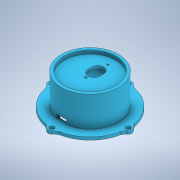
# Autodesk Inventor part: Pieza1parte3
Saved by Autodesk Inventor 2021 (Build 250183000, 183)
## iProperties
Created: 2021-03-28
Part Number: Pieza1parte3
Material: Genérico
Document SubType Name: Modeling
Designer: Arturo
Density: 1 g/cm^3
Appearance: Valor por defecto
Author: Arturo
Autodesk Inventor part; units mm, degrees
ref_plane "YZ Plane" through (0, 0, 0) normal (1, 0, 0) x (0, 1, 0)
ref_plane "XZ Plane" through (0, 0, 0) normal (0, 1, 0) x (-1, 0, 0)
ref_plane "XY Plane" through (0, 0, 0) normal (0, 0, 1) x (1, 0, 0)
sketch "Boceto1" plane through (0, 0, 0) normal (0, 1, 0) x (-1, 0, 0)
  line L0 (0, 0) -> (12.5, 0)
  line L1 (12.5, 0) -> (12.5, -5)
  line L2 (0, -5) -> (0, 0)
  circle A0 centre (6.25, -2.5) radius 1
  arc A1 (8.4861, -5) -> (4.0139, -5) centre (6.25, -7) ccw
  line L3 (12.5, -5) -> (8.4861, -5)
  line L4 (4.0139, -5) -> (0, -5)
  dimension "d1" = 5
  dimension "d2" = 2
  dimension "d4" = 6
  constraints: 10 end point, 3 parallel, 2 centre point, 2 point on circle, 1 horizontal, 1 perpendicular
  measures "d1" distance of L0.end L1.end
  measures "d2" diameter of A0
  measures "d4" diameter of A1
extrude "Extrusión1" add sketch "Boceto1" along normal blind 5
sketch "Boceto2" plane through (0, 5, 0) normal (0, 1, 0) x (1, 0, 0)
  line L0 (0, 5) -> (-4.0139, 5) projected
  arc A0 (-8.4861, 5) -> (-4.0139, 5) centre (-6.25, 7) ccw projected
  line L1 (-8.4861, 5) -> (-12.5, 5) projected
  line L2 (-12.5, 5) -> (-12.5, 0) projected
  line L3 (-12.5, 0) -> (0, 0) projected
  line L4 (0, 0) -> (0, 5) projected
  circle A1 centre (-6.25, 2.5) radius 1 projected
  arc A2 (-12.5, 11.25) -> (0, 11.25) centre (-6.25, 11.25) ccw
  arc A3 (0, 15.25) -> (-12.5, 15.25) centre (-6.25, 15.25) ccw
  line L5 (-12.5, 11.25) -> (-12.5, 15.25)
  line L6 (0, 11.25) -> (0, 15.25)
  line L7 (0, 23.25) -> (-12.5, 23.25)
  line L8 (-12.5, 23.25) -> (-12.5, 28.25)
  line L9 (-12.5, 28.25) -> (0, 28.25)
  line L10 (0, 28.25) -> (0, 23.25)
  circle A4 centre (-6.25, 25.75) radius 1
  circle A5 centre (-6.25, 7) radius 27
  circle A6 centre (-6.25, 7) radius 30
  dimension "d8" = 12.5
  dimension "d10" = 12.5
  dimension "d12" = 12.5
  dimension "d13" = 5
  dimension "d14" = 2
  dimension "d15" = 54
  dimension "d17" = 3
  constraints: 12 end point, 5 centre point, 4 point on circle, 2 coincident, 2 parallel, 2 tangent, 1 horizontal, 1 perpendicular
  measures "d8" diameter of A2
  measures "d10" diameter of A3
  measures "d12" distance of L8.end L9.end
  measures "d13" distance of L7.end L8.end
  measures "d14" diameter of A4
  measures "d15" diameter of A5
  measures "d17" radial gap between concentric circles of A5 A6
extrude "Extrusión2" add sketch "Boceto2" along normal blind 3 contours A5
extrude "Extrusión3" add sketch "Boceto2" against normal blind 5 contours L7 L8 L9 L10
extrude "Extrusión4" add sketch "Boceto2" along normal blind 6.8 contours A6
sketch "Boceto3" plane through (0, 5, 0) normal (0, 1, 0) x (1, 0, 0)
  line L0 (-4.0139, 5) -> (0, 5) projected
  line L1 (0, 0) -> (-12.5, 0) projected
  line L2 (0, 5) -> (-12.5, 5)
  line L3 (-12.5, 5) -> (-12.5, 0)
  line L4 (-12.5, 0) -> (0, 0)
  line L5 (0, 0) -> (0, 5)
  line L6 (-12.5, 28.25) -> (0, 28.25) projected
  line L7 (0, 23.25) -> (-12.5, 23.25) projected
  line L8 (0, 28.25) -> (-12.5, 28.25)
  line L9 (-12.5, 28.25) -> (-12.5, 23.25)
  line L10 (-12.5, 23.25) -> (0, 23.25)
  line L11 (0, 23.25) -> (0, 28.25)
  circle A0 centre (-6.25, 25.75) radius 1 projected
  circle A1 centre (-6.25, 25.75) radius 1
  circle A2 centre (-6.25, 2.5) radius 1 projected
  circle A3 centre (-6.25, 2.5) radius 1
  dimension "d24" = 12.5
  dimension "d25" = 5
  dimension "d26" = 12.5
  dimension "d27" = 5
  dimension "d28" = 2
  dimension "d29" = 2
  constraints: 16 end point, 4 parallel, 2 centre point, 2 coincident, 2 horizontal, 2 perpendicular
  measures "d24" distance of L4.end L1.end
  measures "d25" distance of L1.end L2.end
  measures "d26" distance of L10.end L7.end
  measures "d27" distance of L7.end L8.end
  measures "d28" diameter of A1
  measures "d29" diameter of A3
extrude "Extrusión5" add sketch "Boceto3" along normal blind 3
sketch "Boceto4" plane through (-6.25, 5, -7) normal (0, -1, 0) x (1, 0, 0)
  circle A0 centre (0, 0) radius 27 projected
  circle A1 centre (0, 0) radius 30
  circle A2 centre (0, 0) radius 27
  point P0 (6.25, 7)
  dimension "d32" = 60
  dimension "d33" = 54
  constraints: 2 centre point, 2 coincident
  measures "d32" diameter of A1
  measures "d33" diameter of A2
extrude "Extrusión6" add sketch "Boceto4" along normal blind 25
sketch "Boceto5" plane through (-6.25, -20, -7) normal (0, -1, 0) x (1, 0, 0)
  circle A0 centre (0, 0) radius 27 projected
  arc A1 (6.25, -4.25) -> (-6.25, -4.25) centre (0, -4.25) ccw projected
  line L0 (6.25, -8.25) -> (6.25, -4.25) projected
  arc A2 (-6.25, -8.25) -> (6.25, -8.25) centre (0, -8.25) ccw projected
  line L1 (-6.25, -4.25) -> (-6.25, -8.25) projected
  arc A3 (2.2361, 2) -> (-2.2361, 2) centre (0, 0) ccw projected
  line L2 (-2.2361, 2) -> (-6.25, 2) projected
  line L3 (-6.25, 2) -> (-6.25, 7) projected
  line L4 (-6.25, 7) -> (6.25, 7) projected
  line L5 (6.25, 7) -> (6.25, 2) projected
  line L6 (6.25, 2) -> (2.2361, 2) projected
  line L7 (6.25, -16.25) -> (-6.25, -16.25) projected
  line L8 (6.25, -21.25) -> (6.25, -16.25) projected
  line L9 (-6.25, -21.25) -> (6.25, -21.25) projected
  line L10 (-6.25, -16.25) -> (-6.25, -21.25) projected
  circle A4 centre (0, 0) radius 30 projected
  circle A5 centre (0, 0) radius 27 projected
  circle A6 centre (0, 0) radius 40
  circle A7 centre (0, 0) radius 30 projected
  line L11 (0, 30) -> (5, 30)
  line L12 (5, 30) -> (-5, 30)
  line L13 (-5, 30) -> (-5, 26.533)
  circle A8 centre (0, 0) radius 27 projected
  line L14 (5, 30) -> (5, 26.533)
  circle A9 centre (0, 0) radius 27
  circle A10 centre (0, 0) radius 30
  dimension "d36" = 80
  dimension "d37" = 5
  dimension "d38" = 10
  constraints: 8 end point, 3 centre point, 3 coincident, 2 horizontal, 2 point on circle, 1 concentric, 1 parallel, 1 perpendicular, 1 point on line, 1 vertical alignment, 2 other
  measures "d36" diameter of A6
  measures "d37" distance of L11.start L11.end
  measures "d38" distance of L11.end L12.end
extrude "Extrusión7" add sketch "Boceto5" along normal blind 3 contours A0 L14 A4 L13 | A0 L13 A4 L14 | A4 L11 L14 | L13 L12 A4 | A6
sketch "Boceto6" plane through (-6.25, -23, -7) normal (0, -1, 0) x (1, 0, 0)
  circle A0 centre (0, 0) radius 30 projected
  circle A1 centre (0, 0) radius 40 projected
  circle A2 centre (0, 0) radius 27 projected
  circle A3 centre (0, 0) radius 30 projected
  circle A4 centre (0, 0) radius 30 projected
  circle A5 centre (0, 0) radius 40 projected
  arc A6 (42.4961, -3.1256) -> (42.4568, 3.1566) centre (40, 0) ccw
  circle A7 centre (40, 0) radius 2.5
  circle A8 centre (0, 0) radius 40
  arc A9 (42.4961, -3.1256) -> (39.2164, -7.8789) centre (48.7365, -10.9396) ccw
  line L0 (39.8, 3.995) -> (39.8, 3.995)
  arc A10 (39.3287, 7.2975) -> (42.4568, 3.1566) centre (48.5987, 11.0482) ccw
  arc A11 (3.1545, 42.4596) -> (-3.1252, 42.4966) centre (0, 40) ccw
  circle A12 centre (0, 40) radius 2.5
  line L1 (3.995, 39.8) -> (3.995, 39.8)
  line L2 (9.1155, 38.7955) -> (7.182, 39.1748)
  arc A13 (3.1545, 42.4596) -> (9.1155, 38.7955) centre (11.0406, 48.6084) ccw
  line L3 (-3.995, 39.8) -> (-3.995, 39.8)
  line L4 (-9.2166, 38.8873) -> (-9.7422, 38.7955)
  arc A14 (-9.2166, 38.8873) -> (-3.1252, 42.4966) centre (-10.9383, 48.738) ccw
  arc A15 (-3.2297, -42.3598) -> (3.1372, -42.4816) centre (0, -40) ccw
  circle A16 centre (0, -40) radius 2.5
  arc A17 (-42.4596, 3.1545) -> (-42.4753, -3.1421) centre (-40, 0) ccw
  circle A18 centre (-40, 0) radius 2.5
  line L5 (-8.8392, -38.5679) -> (-8.6091, -38.6265)
  arc A19 (7.6163, -39.2682) -> (3.1372, -42.4816) centre (10.9801, -48.6855) ccw
  arc A20 (-3.2297, -42.3598) -> (-6.5544, -39.4593) centre (-11.3041, -48.2594) ccw
  arc A21 (-42.4596, 3.1545) -> (-39.3229, 7.3286) centre (-48.6084, 11.0406) ccw
  arc A22 (-39.2858, -7.5248) -> (-42.4753, -3.1421) centre (-48.6635, -10.9974) ccw
  point P0 (6.25, 7)
  point P1 (39.8, -3.995)
  point P2 (3.995, -39.8)
  point P3 (-3.995, -39.8)
  point P4 (-39.8, -3.995)
  point P5 (-39.8, 3.995)
  point P6 (-39.2858, -7.5248)
  point P7 (-39.9219, -2.4988)
  point P8 (-39.9219, 2.4988)
  point P9 (-39.3229, 7.3286)
  point P10 (-7.8886, 39.2144)
  point P11 (-2.4988, 39.9219)
  point P12 (2.4988, 39.9219)
  point P13 (7.3286, 39.3229)
  point P14 (2.4988, -39.9219)
  point P15 (-2.4988, -39.9219)
  point P16 (-6.5544, -39.4593)
  point P17 (39.3287, 7.2975)
  point P18 (39.9219, 2.4988)
  point P19 (39.9219, -2.4988)
  dimension "d41" = 8
  dimension "d42" = 5
  dimension "d43" = 10
  dimension "d44" = 10
  dimension "d45" = 8
  dimension "d46" = 5
  dimension "d47" = 10
  dimension "d48" = 10
  dimension "d49" = 8
  dimension "d50" = 5
  dimension "d51" = 8
  dimension "d52" = 5
  dimension "d53" = 10
  dimension "d54" = 10
  constraints: 32 point on circle, 16 centre point, 13 tangent, 12 end point, 5 coincident, 3 point on line, 2 equal radius, 1 horizontal alignment, 30 other
  measures "d41" diameter of A6
  measures "d42" diameter of A7
  measures "d43" radius of A9
  measures "d44" radius of A10
  measures "d45" diameter of A11
  measures "d46" diameter of A12
  measures "d47" radius of A13
  measures "d48" radius of A14
  measures "d49" diameter of A15
  measures "d50" diameter of A16
  measures "d51" diameter of A17
  measures "d52" diameter of A18
  measures "d53" radius of A19
  measures "d54" radius of A21
extrude "Extrusión8" add sketch "Boceto6" against normal blind 3 contours A1 A18 A22 A17 A21 | A14 A11 A13 A1 A12 | A1 A16 A19 A15 A20 | A10 A6 A9 A1 A7
extrude "Extrusión9" cut sketch "Boceto6" against normal blind 3 contours A18 A1 | A1 A12 | A16 A1 | A1 A7 picked at (-39.1609, 0) picked at (-0.0985, 39.1667) picked at (-0.0985, -39.1667) picked at (39.2158, -0.5677)
sketch "Boceto7" plane through (0, 0, 0) normal (0, 0, 1) x (1, 0, 0)
  line L0 (-36.25, -20) -> (23.75, -20) projected
  line L1 (23.75, 11.8) -> (-36.25, 11.8) projected
  line L2 (-3.0955, -23) -> (-9.3752, -23) projected
  line L3 (-3.0955, -23) -> (-3.0955, -20) projected
  line L4 (-9.3752, -20) -> (-3.0955, -20) projected
  line L5 (-9.3752, -23) -> (-9.3752, -20) projected
  line L6 (1.0786, -23) -> (-3.0955, -23) projected
  line L7 (1.0786, -20) -> (1.0786, -23) projected
  line L8 (-3.0955, -20) -> (1.0786, -20) projected
  line L9 (-3.0955, -23) -> (-3.0955, -20) projected
  line L10 (-12.8044, -20) -> (-12.8044, -23) projected
  line L11 (-9.3752, -23) -> (-14.1386, -23) projected
  line L12 (-9.3752, -23) -> (-9.3752, -20) projected
  line L13 (-14.1386, -20) -> (-9.3752, -20) projected
  line L14 (-14.1386, -23) -> (-14.1386, -20) projected
  line L15 (-3.75, -20) -> (-3.75, -23) projected
  line L16 (-3.75, -21.5) -> (-8.75, -21.5)
  line L17 (-6.25, -22.5562) -> (-1.25, -22.5562)
  line L18 (-1.25, -22.5562) -> (-11.25, -22.5562)
  line L19 (-11.25, -22.5562) -> (-11.25, -20)
  line L20 (-11.25, -20) -> (-1.25, -20)
  line L21 (-1.25, -20) -> (-1.25, -15)
  line L22 (-1.25, -15) -> (-11.25, -15)
  line L23 (-11.25, -15) -> (-11.25, -20)
  point P0 (0, 0)
  dimension "d59" = 5
  dimension "d60" = 5
  dimension "d61" = 10
  dimension "d62" = 10
  dimension "d63" = 5
  constraints: 16 end point, 3 parallel, 2 horizontal, 2 perpendicular, 2 point on line, 1 midpoint
  measures "d59" distance of L16.start L16.end
  measures "d60" distance of L17.start L17.end
  measures "d61" distance of L17.end L18.end
  measures "d62" distance of L22.end L21.end
  measures "d63" distance of L21.end L20.end
extrude "Extrusión10" cut sketch "Boceto7" along normal blind 30 contours L23 L22 L21 L0
